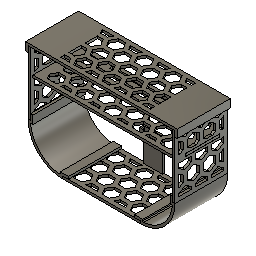
carcasa_abeja v3 (Autodesk Fusion 360 design; units mm, degrees)
Autodesk Fusion 360 part; units mm, degrees
(part 1 of 3)
sketch "Boceto1" plane through (0, 0, 0) normal (0, 1, 0) x (1, 0, 0)
  line L0 (0, 0) -> (1800, 0)
  line L1 (1800, 0) -> (1800, -650)
  line L2 (1800, -650) -> (0, -650)
  line L3 (0, -650) -> (0, 0)
  dimension "d1" = 650
  dimension "d2" = 1800
  constraint horizontal L0
  constraint vertical L1
  constraint horizontal L2
  constraint vertical L3
  constraint coincident L0.start L3.end
  measures "d1" distance of L0.end L1.end
  measures "d2" distance of L1.end L2.end
extrude "Extruir1" add sketch "Boceto1" along normal blind 30 makes body 1
sketch "Boceto3" plane through (0, 0, 0) normal (0, -1, 0) x (1, 0, 0)
  line L0 (0, 650) -> (0, 0)
  line L1 (0, 0) -> (1800, 0) construction
  line L2 (1800, 0) -> (1800, 650)
  line L3 (50, 50) -> (1750, 50)
  line L4 (1750, 50) -> (1750, 600)
  line L5 (1750, 600) -> (50, 600)
  line L6 (50, 600) -> (50, 50)
  line L7 (900, 50) -> (900, 600) construction
  line L8 (986.6025, 325) -> (943.3013, 400)
  line L9 (943.3013, 400) -> (856.6987, 400)
  line L10 (856.6987, 400) -> (813.3975, 325)
  line L11 (813.3975, 325) -> (856.6987, 250)
  line L12 (856.6987, 250) -> (943.3013, 250)
  line L13 (943.3013, 250) -> (986.6025, 325)
  line L14 (900, 325) -> (964.9519, 362.5) construction
  line L15 (1636.1216, 0) -> (1549.5191, 0) construction
  line L16 (1722.7241, 100) -> (1693.8566, 50)
  line L17 (1289.7114, 0) -> (1203.1089, 0) construction
  line L18 (1491.784, 50) -> (1462.9165, 100)
  line L19 (1376.314, 100) -> (1347.4465, 50)
  line L20 (1462.9165, 100) -> (1376.314, 100)
  line L21 (1506.2178, 125) -> (1549.5191, 50)
  line L22 (1549.5191, 50) -> (1636.1216, 50) construction
  line L23 (1636.1216, 50) -> (1679.4229, 125)
  line L24 (1679.4229, 125) -> (1636.1216, 200)
  line L25 (1549.5191, 200) -> (1506.2178, 125)
  line L26 (1636.1216, 200) -> (1549.5191, 200)
  line L27 (1679.4229, 225) -> (1722.7241, 150)
  line L28 (1722.7241, 300) -> (1679.4229, 225)
  line L29 (943.3013, 0) -> (856.6987, 0) construction
  line L30 (1145.3739, 50) -> (1116.5064, 100)
  line L31 (1029.9038, 100) -> (1001.0363, 50)
  line L32 (1116.5064, 100) -> (1029.9038, 100)
  line L33 (1159.8076, 125) -> (1203.1089, 50)
  line L34 (1203.1089, 50) -> (1289.7114, 50) construction
  line L35 (1289.7114, 50) -> (1333.0127, 125)
  line L36 (1333.0127, 125) -> (1289.7114, 200)
  line L37 (1203.1089, 200) -> (1159.8076, 125)
  line L38 (1289.7114, 200) -> (1203.1089, 200)
  line L39 (1333.0127, 225) -> (1376.314, 150)
  line L40 (1376.314, 150) -> (1462.9165, 150)
  line L41 (1462.9165, 150) -> (1506.2178, 225)
  line L42 (1506.2178, 225) -> (1462.9165, 300)
  line L43 (1376.314, 300) -> (1333.0127, 225)
  line L44 (1462.9165, 300) -> (1376.314, 300)
  line L45 (1506.2178, 325) -> (1549.5191, 250)
  line L46 (1549.5191, 250) -> (1636.1216, 250)
  line L47 (1636.1216, 250) -> (1679.4229, 325)
  line L48 (1679.4229, 325) -> (1636.1216, 400)
  line L49 (1549.5191, 400) -> (1506.2178, 325)
  line L50 (1636.1216, 400) -> (1549.5191, 400)
  line L51 (1679.4229, 425) -> (1722.7241, 350)
  line L52 (1722.7241, 500) -> (1679.4229, 425)
  line L53 (596.8911, 0) -> (510.2886, 0) construction
  line L54 (798.9637, 50) -> (770.0962, 100)
  line L55 (683.4936, 100) -> (654.6261, 50)
  line L56 (770.0962, 100) -> (683.4936, 100)
  line L57 (813.3975, 125) -> (856.6987, 50)
  line L58 (856.6987, 50) -> (943.3013, 50) construction
  line L59 (943.3013, 50) -> (986.6025, 125)
  line L60 (986.6025, 125) -> (943.3013, 200)
  line L61 (856.6987, 200) -> (813.3975, 125)
  line L62 (943.3013, 200) -> (856.6987, 200)
  line L63 (986.6025, 225) -> (1029.9038, 150)
  line L64 (1029.9038, 150) -> (1116.5064, 150)
  line L65 (1116.5064, 150) -> (1159.8076, 225)
  line L66 (1159.8076, 225) -> (1116.5064, 300)
  line L67 (1029.9038, 300) -> (986.6025, 225)
  line L68 (1116.5064, 300) -> (1029.9038, 300)
  line L69 (1159.8076, 325) -> (1203.1089, 250)
  line L70 (1203.1089, 250) -> (1289.7114, 250)
  line L71 (1289.7114, 250) -> (1333.0127, 325)
  line L72 (1333.0127, 325) -> (1289.7114, 400)
  line L73 (1203.1089, 400) -> (1159.8076, 325)
  line L74 (1289.7114, 400) -> (1203.1089, 400)
  line L75 (1333.0127, 425) -> (1376.314, 350)
  line L76 (1376.314, 350) -> (1462.9165, 350)
  line L77 (1462.9165, 350) -> (1506.2178, 425)
  line L78 (1506.2178, 425) -> (1462.9165, 500)
  line L79 (1376.314, 500) -> (1333.0127, 425)
  line L80 (1462.9165, 500) -> (1376.314, 500)
  line L81 (1506.2178, 525) -> (1549.5191, 450)
  line L82 (1549.5191, 450) -> (1636.1216, 450)
  line L83 (1636.1216, 450) -> (1679.4229, 525)
  line L84 (1679.4229, 525) -> (1636.1216, 600)
  line L85 (1549.5191, 600) -> (1506.2178, 525)
  line L86 (1636.1216, 600) -> (1549.5191, 600)
  line L87 (1693.8566, 600) -> (1722.7241, 550)
  line L88 (250.4809, 0) -> (163.8784, 0) construction
  line L89 (452.5535, 50) -> (423.686, 100)
  line L90 (337.0835, 100) -> (308.216, 50)
  line L91 (423.686, 100) -> (337.0835, 100)
  line L92 (466.9873, 125) -> (510.2886, 50)
  line L93 (510.2886, 50) -> (596.8911, 50) construction
  line L94 (596.8911, 50) -> (640.1924, 125)
  line L95 (640.1924, 125) -> (596.8911, 200)
  line L96 (510.2886, 200) -> (466.9873, 125)
  line L97 (596.8911, 200) -> (510.2886, 200)
  line L98 (640.1924, 225) -> (683.4936, 150)
  line L99 (683.4936, 150) -> (770.0962, 150)
  line L100 (770.0962, 150) -> (813.3975, 225)
  line L101 (813.3975, 225) -> (770.0962, 300)
  line L102 (683.4936, 300) -> (640.1924, 225)
  line L103 (770.0962, 300) -> (683.4936, 300)
  line L104 (986.6025, 425) -> (1029.9038, 350)
  line L105 (1029.9038, 350) -> (1116.5064, 350)
  line L106 (1116.5064, 350) -> (1159.8076, 425)
  line L107 (1159.8076, 425) -> (1116.5064, 500)
  line L108 (1029.9038, 500) -> (986.6025, 425)
  line L109 (1116.5064, 500) -> (1029.9038, 500)
  line L110 (1159.8076, 525) -> (1203.1089, 450)
  line L111 (1203.1089, 450) -> (1289.7114, 450)
  line L112 (1289.7114, 450) -> (1333.0127, 525)
  line L113 (1333.0127, 525) -> (1289.7114, 600)
  line L114 (1203.1089, 600) -> (1159.8076, 525)
  line L115 (1289.7114, 600) -> (1203.1089, 600)
  line L116 (1347.4465, 600) -> (1376.314, 550)
  line L117 (1376.314, 550) -> (1462.9165, 550)
  line L118 (1462.9165, 550) -> (1491.784, 600)
  line L119 (106.1434, 50) -> (77.2759, 100)
  line L120 (120.5771, 125) -> (163.8784, 50)
  line L121 (163.8784, 50) -> (250.4809, 50) construction
  line L122 (250.4809, 50) -> (293.7822, 125)
  line L123 (293.7822, 125) -> (250.4809, 200)
  line L124 (163.8784, 200) -> (120.5771, 125)
  line L125 (250.4809, 200) -> (163.8784, 200)
  line L126 (293.7822, 225) -> (337.0835, 150)
  line L127 (337.0835, 150) -> (423.686, 150)
  line L128 (423.686, 150) -> (466.9873, 225)
  line L129 (466.9873, 225) -> (423.686, 300)
  line L130 (337.0835, 300) -> (293.7822, 225)
  line L131 (423.686, 300) -> (337.0835, 300)
  line L132 (466.9873, 325) -> (510.2886, 250)
  line L133 (510.2886, 250) -> (596.8911, 250)
  line L134 (596.8911, 250) -> (640.1924, 325)
  line L135 (640.1924, 325) -> (596.8911, 400)
  line L136 (510.2886, 400) -> (466.9873, 325)
  line L137 (596.8911, 400) -> (510.2886, 400)
  line L138 (640.1924, 425) -> (683.4936, 350)
  line L139 (683.4936, 350) -> (770.0962, 350)
  line L140 (770.0962, 350) -> (813.3975, 425)
  line L141 (813.3975, 425) -> (770.0962, 500)
  line L142 (683.4936, 500) -> (640.1924, 425)
  line L143 (770.0962, 500) -> (683.4936, 500)
  line L144 (813.3975, 525) -> (856.6987, 450)
  line L145 (856.6987, 450) -> (943.3013, 450)
  line L146 (943.3013, 450) -> (986.6025, 525)
  line L147 (986.6025, 525) -> (943.3013, 600)
  line L148 (856.6987, 600) -> (813.3975, 525)
  line L149 (943.3013, 600) -> (856.6987, 600)
  line L150 (1001.0363, 600) -> (1029.9038, 550)
  line L151 (1029.9038, 550) -> (1116.5064, 550)
  line L152 (1116.5064, 550) -> (1145.3739, 600)
  line L153 (77.2759, 150) -> (120.5771, 225)
  line L154 (120.5771, 225) -> (77.2759, 300)
  line L155 (120.5771, 325) -> (163.8784, 250)
  line L156 (163.8784, 250) -> (250.4809, 250)
  line L157 (250.4809, 250) -> (293.7822, 325)
  line L158 (293.7822, 325) -> (250.4809, 400)
  line L159 (163.8784, 400) -> (120.5771, 325)
  line L160 (250.4809, 400) -> (163.8784, 400)
  line L161 (293.7822, 425) -> (337.0835, 350)
  line L162 (337.0835, 350) -> (423.686, 350)
  line L163 (423.686, 350) -> (466.9873, 425)
  line L164 (466.9873, 425) -> (423.686, 500)
  line L165 (337.0835, 500) -> (293.7822, 425)
  line L166 (423.686, 500) -> (337.0835, 500)
  line L167 (466.9873, 525) -> (510.2886, 450)
  line L168 (510.2886, 450) -> (596.8911, 450)
  line L169 (596.8911, 450) -> (640.1924, 525)
  line L170 (640.1924, 525) -> (596.8911, 600)
  line L171 (510.2886, 600) -> (466.9873, 525)
  line L172 (596.8911, 600) -> (510.2886, 600)
  line L173 (654.6261, 600) -> (683.4936, 550)
  line L174 (683.4936, 550) -> (770.0962, 550)
  line L175 (770.0962, 550) -> (798.9637, 600)
  line L176 (77.2759, 350) -> (120.5771, 425)
  line L177 (120.5771, 425) -> (77.2759, 500)
  line L178 (120.5771, 525) -> (163.8784, 450)
  line L179 (163.8784, 450) -> (250.4809, 450)
  line L180 (250.4809, 450) -> (293.7822, 525)
  line L181 (293.7822, 525) -> (250.4809, 600)
  line L182 (163.8784, 600) -> (120.5771, 525)
  line L183 (250.4809, 600) -> (163.8784, 600)
  line L184 (308.216, 600) -> (337.0835, 550)
  line L185 (337.0835, 550) -> (423.686, 550)
  line L186 (423.686, 550) -> (452.5535, 600)
  line L187 (77.2759, 550) -> (106.1434, 600)
  line L188 (77.2759, 500) -> (50, 500)
  line L189 (0, 500) -> (-9.3267, 500)
  line L190 (-9.3267, 350) -> (0, 350)
  line L191 (50, 350) -> (77.2759, 350)
  line L192 (-9.3267, 550) -> (0, 550)
  line L193 (50, 550) -> (77.2759, 550)
  line L194 (1722.7241, 550) -> (1750, 550)
  line L195 (1800, 550) -> (1809.3267, 550)
  line L196 (1809.3267, 500) -> (1800, 500)
  line L197 (1750, 500) -> (1722.7241, 500)
  line L198 (1722.7241, 350) -> (1750, 350)
  line L199 (1800, 350) -> (1809.3267, 350)
  line L200 (1809.3267, 300) -> (1800, 300)
  line L201 (1750, 300) -> (1722.7241, 300)
  line L202 (1722.7241, 150) -> (1750, 150)
  line L203 (1800, 150) -> (1809.3267, 150)
  line L204 (1809.3267, 100) -> (1800, 100)
  line L205 (1750, 100) -> (1722.7241, 100)
  line L206 (77.2759, 100) -> (50, 100)
  line L207 (0, 100) -> (-9.3267, 100)
  line L208 (-9.3267, 150) -> (0, 150)
  line L209 (50, 150) -> (77.2759, 150)
  line L210 (77.2759, 300) -> (50, 300)
  line L211 (0, 300) -> (-9.3267, 300)
  point P0 (900, 325)
  dimension "d15" = 200
  dimension "d16" = 200
  dimension "d17" = 150
  constraint midpoint L3 L7.start
  constraint midpoint L5 L7.end
  constraint midpoint L7 P0
  constraint parallel L3 L12
  constraint coincident P0 L14.start
  constraint midpoint L8 L14.end
  constraint coincident L6 L188.end
  constraint coincident L0 L189.start
  constraint collinear L188 L189
  constraint coincident L0 L190.end
  constraint coincident L6 L191.start
  constraint collinear L190 L191
  constraint coincident L0 L192.end
  constraint coincident L6 L193.start
  constraint collinear L192 L193
  constraint coincident L5 L187.end
  constraint coincident L5 L184.start
  constraint coincident L5 L186.end
  constraint coincident L5 L173.start
  constraint coincident L5 L175.end
  constraint coincident L5 L150.start
  constraint coincident L5 L152.end
  constraint coincident L5 L116.start
  constraint coincident L5 L118.end
  constraint coincident L5 L87.start
  constraint coincident L4 L194.end
  constraint coincident L2 L195.start
  constraint collinear L194 L195
  constraint coincident L2 L196.end
  constraint coincident L4 L197.start
  constraint collinear L196 L197
  constraint coincident L4 L198.end
  constraint coincident L2 L199.start
  constraint collinear L198 L199
  constraint coincident L2 L200.end
  constraint coincident L4 L201.start
  constraint collinear L200 L201
  constraint coincident L4 L202.end
  constraint coincident L2 L203.start
  constraint collinear L202 L203
  constraint coincident L2 L204.end
  constraint coincident L4 L205.start
  constraint collinear L204 L205
  constraint coincident L3 L16.end
  constraint coincident L3 L18.start
  constraint coincident L3 L19.end
  constraint coincident L3 L30.start
  constraint coincident L3 L31.end
  constraint coincident L3 L54.start
  constraint coincident L3 L55.end
  constraint coincident L3 L89.start
  constraint coincident L3 L90.end
  constraint coincident L3 L119.start
  constraint coincident L6 L206.end
  constraint coincident L0 L207.start
  constraint collinear L206 L207
  constraint coincident L0 L208.end
  constraint coincident L6 L209.start
  constraint collinear L208 L209
  constraint coincident L6 L210.end
  constraint coincident L0 L211.start
  constraint collinear L210 L211
  measures "d17" distance of L8.end L12.end
extrude "Extruir2" cut sketch "Boceto3" against normal blind 300 contours L3 L6 L119 L206 | L3 L120 L122 L123 L124 L125 | L6 L153 L154 L209 L210 | L3 L89 L90 L91 | L6 L176 L177 L188 L191 | L3 L92 L94 L95 L96 L97 | L5 L6 L187 L193 | L3 L54 L55 L56 | L5 L178 L179 L180 L181 L182 L183 | L3 L57 L59 L60 L61 L62 | L5 L184 L185 L186 | L3 L30 L31 L32 | L5 L167 L168 L169 L170 L171 L172 | L3 L33 L35 L36 L37 L38 | L5 L173 L174 L175 | L3 L18 L19 L20 | L5 L144 L145 L146 L147 L148 L149 | L3 L21 L23 L24 L25 L26 | L5 L150 L151 L152 | L3 L4 L16 L205 | L5 L110 L111 L112 L113 L114 L115 | L4 L27 L28 L201 L202 | L5 L116 L117 L118 | L4 L51 L52 L197 L198 | L5 L81 L82 L83 L84 L85 L86 | L4 L5 L87 L194 | L8 L9 L10 L11 L12 L13 | L39 L40 L41 L42 L43 L44 | L45 L46 L47 L48 L49 L50 | L63 L64 L65 L66 L67 L68 | L69 L70 L71 L72 L73 L74 | L75 L76 L77 L78 L79 L80 | L98 L99 L100 L101 L102 L103 | L104 L105 L106 L107 L108 L109 | L126 L127 L128 L129 L130 L131 | L132 L133 L134 L135 L136 L137 | L138 L139 L140 L141 L142 L143 | L155 L156 L157 L158 L159 L160 | L161 L162 L163 L164 L165 L166 bodies 1
sketch "Boceto4" plane through (0, 30, 0) normal (0, 1, 0) x (-1, 0, 0)
  line L0 (-1549.5191, 200) -> (-1506.2178, 125)
  line L1 (-1506.2178, 125) -> (-1549.5191, 50)
  line L2 (-1549.5191, 50) -> (-1636.1216, 50)
  line L3 (-1636.1216, 50) -> (-1679.4229, 125)
  line L4 (-1679.4229, 125) -> (-1636.1216, 200)
  line L5 (-1636.1216, 200) -> (-1549.5191, 200)
  line L6 (-1750, 550) -> (-1750, 600)
  line L7 (-1750, 600) -> (-1693.8566, 600)
  line L8 (-1693.8566, 600) -> (-1722.7241, 550)
  line L9 (-1722.7241, 550) -> (-1750, 550)
  line L10 (-1376.314, 300) -> (-1333.0127, 225)
  line L11 (-1333.0127, 225) -> (-1376.314, 150)
  line L12 (-1376.314, 150) -> (-1462.9165, 150)
  line L13 (-1462.9165, 150) -> (-1506.2178, 225)
  line L14 (-1506.2178, 225) -> (-1462.9165, 300)
  line L15 (-1462.9165, 300) -> (-1376.314, 300)
  line L16 (-1203.1089, 600) -> (-1159.8076, 525)
  line L17 (-1159.8076, 525) -> (-1203.1089, 450)
  line L18 (-1203.1089, 450) -> (-1289.7114, 450)
  line L19 (-1289.7114, 450) -> (-1333.0127, 525)
  line L20 (-1333.0127, 525) -> (-1289.7114, 600)
  line L21 (-1289.7114, 600) -> (-1203.1089, 600)
  line L22 (-856.6987, 200) -> (-813.3975, 125)
  line L23 (-813.3975, 125) -> (-856.6987, 50)
  line L24 (-856.6987, 50) -> (-943.3013, 50)
  line L25 (-943.3013, 50) -> (-986.6025, 125)
  line L26 (-986.6025, 125) -> (-943.3013, 200)
  line L27 (-943.3013, 200) -> (-856.6987, 200)
  line L28 (-856.6987, 600) -> (-813.3975, 525)
  line L29 (-813.3975, 525) -> (-856.6987, 450)
  line L30 (-856.6987, 450) -> (-943.3013, 450)
  line L31 (-943.3013, 450) -> (-986.6025, 525)
  line L32 (-986.6025, 525) -> (-943.3013, 600)
  line L33 (-943.3013, 600) -> (-856.6987, 600)
  line L34 (-510.2886, 400) -> (-466.9873, 325)
  line L35 (-466.9873, 325) -> (-510.2886, 250)
  line L36 (-510.2886, 250) -> (-596.8911, 250)
  line L37 (-596.8911, 250) -> (-640.1924, 325)
  line L38 (-640.1924, 325) -> (-596.8911, 400)
  line L39 (-596.8911, 400) -> (-510.2886, 400)
  line L40 (-163.8784, 400) -> (-120.5771, 325)
  line L41 (-120.5771, 325) -> (-163.8784, 250)
  line L42 (-163.8784, 250) -> (-250.4809, 250)
  line L43 (-250.4809, 250) -> (-293.7822, 325)
  line L44 (-293.7822, 325) -> (-250.4809, 400)
  line L45 (-250.4809, 400) -> (-163.8784, 400)
  line L46 (-77.2759, 350) -> (-120.5771, 425)
  line L47 (-120.5771, 425) -> (-77.2759, 500)
  line L48 (-77.2759, 500) -> (-50, 500)
  line L49 (-50, 500) -> (-50, 350)
  line L50 (-50, 350) -> (-77.2759, 350)
  line L51 (-163.8784, 600) -> (-120.5771, 525)
  line L52 (-120.5771, 525) -> (-163.8784, 450)
  line L53 (-163.8784, 450) -> (-250.4809, 450)
  line L54 (-250.4809, 450) -> (-293.7822, 525)
  line L55 (-293.7822, 525) -> (-250.4809, 600)
  line L56 (-250.4809, 600) -> (-163.8784, 600)
  line L57 (-77.2759, 550) -> (-106.1434, 600)
  line L58 (-106.1434, 600) -> (-50, 600)
  line L59 (-50, 600) -> (-50, 550)
  line L60 (-50, 550) -> (-77.2759, 550)
  line L61 (-163.8784, 200) -> (-120.5771, 125)
  line L62 (-120.5771, 125) -> (-163.8784, 50)
  line L63 (-163.8784, 50) -> (-250.4809, 50)
  line L64 (-250.4809, 50) -> (-293.7822, 125)
  line L65 (-293.7822, 125) -> (-250.4809, 200)
  line L66 (-250.4809, 200) -> (-163.8784, 200)
  line L67 (-510.2886, 200) -> (-466.9873, 125)
  line L68 (-466.9873, 125) -> (-510.2886, 50)
  line L69 (-510.2886, 50) -> (-596.8911, 50)
  line L70 (-596.8911, 50) -> (-640.1924, 125)
  line L71 (-640.1924, 125) -> (-596.8911, 200)
  line L72 (-596.8911, 200) -> (-510.2886, 200)
  line L73 (-683.4936, 500) -> (-640.1924, 425)
  line L74 (-640.1924, 425) -> (-683.4936, 350)
  line L75 (-683.4936, 350) -> (-770.0962, 350)
  line L76 (-770.0962, 350) -> (-813.3975, 425)
  line L77 (-813.3975, 425) -> (-770.0962, 500)
  line L78 (-770.0962, 500) -> (-683.4936, 500)
  line L79 (-683.4936, 100) -> (-654.6261, 50)
  line L80 (-654.6261, 50) -> (-798.9637, 50)
  line L81 (-798.9637, 50) -> (-770.0962, 100)
  line L82 (-770.0962, 100) -> (-683.4936, 100)
  line L83 (-1145.3739, 600) -> (-1001.0363, 600)
  line L84 (-1001.0363, 600) -> (-1029.9038, 550)
  line L85 (-1029.9038, 550) -> (-1116.5064, 550)
  line L86 (-1116.5064, 550) -> (-1145.3739, 600)
  line L87 (-1203.1089, 200) -> (-1159.8076, 125)
  line L88 (-1159.8076, 125) -> (-1203.1089, 50)
  line L89 (-1203.1089, 50) -> (-1289.7114, 50)
  line L90 (-1289.7114, 50) -> (-1333.0127, 125)
  line L91 (-1333.0127, 125) -> (-1289.7114, 200)
  line L92 (-1289.7114, 200) -> (-1203.1089, 200)
  line L93 (-1549.5191, 600) -> (-1506.2178, 525)
  line L94 (-1506.2178, 525) -> (-1549.5191, 450)
  line L95 (-1549.5191, 450) -> (-1636.1216, 450)
  line L96 (-1636.1216, 450) -> (-1679.4229, 525)
  line L97 (-1679.4229, 525) -> (-1636.1216, 600)
  line L98 (-1636.1216, 600) -> (-1549.5191, 600)
  line L99 (-1376.314, 100) -> (-1347.4465, 50)
  line L100 (-1347.4465, 50) -> (-1491.784, 50)
  line L101 (-1491.784, 50) -> (-1462.9165, 100)
  line L102 (-1462.9165, 100) -> (-1376.314, 100)
  line L103 (-1750, 150) -> (-1750, 300)
  line L104 (-1750, 300) -> (-1722.7241, 300)
  line L105 (-1722.7241, 300) -> (-1679.4229, 225)
  line L106 (-1679.4229, 225) -> (-1722.7241, 150)
  line L107 (-1722.7241, 150) -> (-1750, 150)
  line L108 (-1750, 350) -> (-1750, 500)
  line L109 (-1750, 500) -> (-1722.7241, 500)
  line L110 (-1722.7241, 500) -> (-1679.4229, 425)
  line L111 (-1679.4229, 425) -> (-1722.7241, 350)
  line L112 (-1722.7241, 350) -> (-1750, 350)
  line L113 (-1376.314, 500) -> (-1333.0127, 425)
  line L114 (-1333.0127, 425) -> (-1376.314, 350)
  line L115 (-1376.314, 350) -> (-1462.9165, 350)
  line L116 (-1462.9165, 350) -> (-1506.2178, 425)
  line L117 (-1506.2178, 425) -> (-1462.9165, 500)
  line L118 (-1462.9165, 500) -> (-1376.314, 500)
  line L119 (-1203.1089, 400) -> (-1159.8076, 325)
  line L120 (-1159.8076, 325) -> (-1203.1089, 250)
  line L121 (-1203.1089, 250) -> (-1289.7114, 250)
  line L122 (-1289.7114, 250) -> (-1333.0127, 325)
  line L123 (-1333.0127, 325) -> (-1289.7114, 400)
  line L124 (-1289.7114, 400) -> (-1203.1089, 400)
  line L125 (-1029.9038, 300) -> (-986.6025, 225)
  line L126 (-986.6025, 225) -> (-1029.9038, 150)
  line L127 (-1029.9038, 150) -> (-1116.5064, 150)
  line L128 (-1116.5064, 150) -> (-1159.8076, 225)
  line L129 (-1159.8076, 225) -> (-1116.5064, 300)
  line L130 (-1116.5064, 300) -> (-1029.9038, 300)
  line L131 (-683.4936, 300) -> (-640.1924, 225)
  line L132 (-640.1924, 225) -> (-683.4936, 150)
  line L133 (-683.4936, 150) -> (-770.0962, 150)
  line L134 (-770.0962, 150) -> (-813.3975, 225)
  line L135 (-813.3975, 225) -> (-770.0962, 300)
  line L136 (-770.0962, 300) -> (-683.4936, 300)
  line L137 (-510.2886, 600) -> (-466.9873, 525)
  line L138 (-466.9873, 525) -> (-510.2886, 450)
  line L139 (-510.2886, 450) -> (-596.8911, 450)
  line L140 (-596.8911, 450) -> (-640.1924, 525)
  line L141 (-640.1924, 525) -> (-596.8911, 600)
  line L142 (-596.8911, 600) -> (-510.2886, 600)
  line L143 (-337.0835, 300) -> (-293.7822, 225)
  line L144 (-293.7822, 225) -> (-337.0835, 150)
  line L145 (-337.0835, 150) -> (-423.686, 150)
  line L146 (-423.686, 150) -> (-466.9873, 225)
  line L147 (-466.9873, 225) -> (-423.686, 300)
  line L148 (-423.686, 300) -> (-337.0835, 300)
  line L149 (-50, 300) -> (-50, 150)
  line L150 (-50, 150) -> (-77.2759, 150)
  line L151 (-77.2759, 150) -> (-120.5771, 225)
  line L152 (-120.5771, 225) -> (-77.2759, 300)
  line L153 (-77.2759, 300) -> (-50, 300)
  line L154 (-337.0835, 500) -> (-293.7822, 425)
  line L155 (-293.7822, 425) -> (-337.0835, 350)
  line L156 (-337.0835, 350) -> (-423.686, 350)
  line L157 (-423.686, 350) -> (-466.9873, 425)
  line L158 (-466.9873, 425) -> (-423.686, 500)
  line L159 (-423.686, 500) -> (-337.0835, 500)
  line L160 (-452.5535, 600) -> (-308.216, 600)
  line L161 (-308.216, 600) -> (-337.0835, 550)
  line L162 (-337.0835, 550) -> (-423.686, 550)
  line L163 (-423.686, 550) -> (-452.5535, 600)
  line L164 (-50, 100) -> (-50, 50)
  line L165 (-50, 50) -> (-106.1434, 50)
  line L166 (-106.1434, 50) -> (-77.2759, 100)
  line L167 (-77.2759, 100) -> (-50, 100)
  line L168 (-337.0835, 100) -> (-308.216, 50)
  line L169 (-308.216, 50) -> (-452.5535, 50)
  line L170 (-452.5535, 50) -> (-423.686, 100)
  line L171 (-423.686, 100) -> (-337.0835, 100)
  line L172 (-798.9637, 600) -> (-654.6261, 600)
  line L173 (-654.6261, 600) -> (-683.4936, 550)
  line L174 (-683.4936, 550) -> (-770.0962, 550)
  line L175 (-770.0962, 550) -> (-798.9637, 600)
  line L176 (-986.6025, 325) -> (-943.3013, 400)
  line L177 (-943.3013, 400) -> (-856.6987, 400)
  line L178 (-856.6987, 400) -> (-813.3975, 325)
  line L179 (-813.3975, 325) -> (-856.6987, 250)
  line L180 (-856.6987, 250) -> (-943.3013, 250)
  line L181 (-943.3013, 250) -> (-986.6025, 325)
  line L182 (-1029.9038, 500) -> (-986.6025, 425)
  line L183 (-986.6025, 425) -> (-1029.9038, 350)
  line L184 (-1029.9038, 350) -> (-1116.5064, 350)
  line L185 (-1116.5064, 350) -> (-1159.8076, 425)
  line L186 (-1159.8076, 425) -> (-1116.5064, 500)
  line L187 (-1116.5064, 500) -> (-1029.9038, 500)
  line L188 (-1029.9038, 100) -> (-1001.0363, 50)
  line L189 (-1001.0363, 50) -> (-1145.3739, 50)
  line L190 (-1145.3739, 50) -> (-1116.5064, 100)
  line L191 (-1116.5064, 100) -> (-1029.9038, 100)
  line L192 (-1491.784, 600) -> (-1347.4465, 600)
  line L193 (-1347.4465, 600) -> (-1376.314, 550)
  line L194 (-1376.314, 550) -> (-1462.9165, 550)
  line L195 (-1462.9165, 550) -> (-1491.784, 600)
  line L196 (-1549.5191, 400) -> (-1506.2178, 325)
  line L197 (-1506.2178, 325) -> (-1549.5191, 250)
  line L198 (-1549.5191, 250) -> (-1636.1216, 250)
  line L199 (-1636.1216, 250) -> (-1679.4229, 325)
  line L200 (-1679.4229, 325) -> (-1636.1216, 400)
  line L201 (-1636.1216, 400) -> (-1549.5191, 400)
  line L202 (-1722.7241, 100) -> (-1693.8566, 50)
  line L203 (-1693.8566, 50) -> (-1750, 50)
  line L204 (-1750, 50) -> (-1750, 100)
  line L205 (-1750, 100) -> (-1722.7241, 100)
  line L206 (0, 650) -> (-1800, 650)
  line L207 (-1800, 650) -> (-1800, 0)
  line L208 (-1800, 0) -> (0, 0)
  line L209 (0, 0) -> (0, 650)
scale "Escala1" factor 0.1 about (986.6025, 30, 325) bodies 1
sketch "Boceto5" plane through (0, 30, 0) normal (0, 1, 0) x (-1, 0, 0)
  line L0 (-1042.8942, 312.5) -> (-1038.5641, 305)
  line L1 (-1038.5641, 305) -> (-1042.8942, 297.5)
  line L2 (-1042.8942, 297.5) -> (-1051.5544, 297.5)
  line L3 (-1051.5544, 297.5) -> (-1055.8846, 305)
  line L4 (-1055.8846, 305) -> (-1051.5544, 312.5)
  line L5 (-1051.5544, 312.5) -> (-1042.8942, 312.5)
  line L6 (-1062.9423, 347.5) -> (-1062.9423, 352.5)
  line L7 (-1062.9423, 352.5) -> (-1057.3279, 352.5)
  line L8 (-1057.3279, 352.5) -> (-1060.2147, 347.5)
  line L9 (-1060.2147, 347.5) -> (-1062.9423, 347.5)
  line L10 (-1025.5737, 322.5) -> (-1021.2436, 315)
  line L11 (-1021.2436, 315) -> (-1025.5737, 307.5)
  line L12 (-1025.5737, 307.5) -> (-1034.2339, 307.5)
  line L13 (-1034.2339, 307.5) -> (-1038.5641, 315)
  line L14 (-1038.5641, 315) -> (-1034.2339, 322.5)
  line L15 (-1034.2339, 322.5) -> (-1025.5737, 322.5)
  line L16 (-1008.2532, 352.5) -> (-1003.923, 345)
  line L17 (-1003.923, 345) -> (-1008.2532, 337.5)
  line L18 (-1008.2532, 337.5) -> (-1016.9134, 337.5)
  line L19 (-1016.9134, 337.5) -> (-1021.2436, 345)
  line L20 (-1021.2436, 345) -> (-1016.9134, 352.5)
  line L21 (-1016.9134, 352.5) -> (-1008.2532, 352.5)
  line L22 (-973.6122, 312.5) -> (-969.282, 305)
  line L23 (-969.282, 305) -> (-973.6122, 297.5)
  line L24 (-973.6122, 297.5) -> (-982.2724, 297.5)
  line L25 (-982.2724, 297.5) -> (-986.6025, 305)
  line L26 (-986.6025, 305) -> (-982.2724, 312.5)
  line L27 (-982.2724, 312.5) -> (-973.6122, 312.5)
  line L28 (-973.6122, 352.5) -> (-969.282, 345)
  line L29 (-969.282, 345) -> (-973.6122, 337.5)
  line L30 (-973.6122, 337.5) -> (-982.2724, 337.5)
  line L31 (-982.2724, 337.5) -> (-986.6025, 345)
  line L32 (-986.6025, 345) -> (-982.2724, 352.5)
  line L33 (-982.2724, 352.5) -> (-973.6122, 352.5)
  line L34 (-938.9711, 332.5) -> (-934.641, 325)
  line L35 (-934.641, 325) -> (-938.9711, 317.5)
  line L36 (-938.9711, 317.5) -> (-947.6314, 317.5)
  line L37 (-947.6314, 317.5) -> (-951.9615, 325)
  line L38 (-951.9615, 325) -> (-947.6314, 332.5)
  line L39 (-947.6314, 332.5) -> (-938.9711, 332.5)
  line L40 (-904.3301, 332.5) -> (-900, 325)
  line L41 (-900, 325) -> (-904.3301, 317.5)
  line L42 (-904.3301, 317.5) -> (-912.9904, 317.5)
  line L43 (-912.9904, 317.5) -> (-917.3205, 325)
  line L44 (-917.3205, 325) -> (-912.9904, 332.5)
  line L45 (-912.9904, 332.5) -> (-904.3301, 332.5)
  line L46 (-895.6699, 327.5) -> (-900, 335)
  line L47 (-900, 335) -> (-895.6699, 342.5)
  line L48 (-895.6699, 342.5) -> (-892.9423, 342.5)
  line L49 (-892.9423, 342.5) -> (-892.9423, 327.5)
  line L50 (-892.9423, 327.5) -> (-895.6699, 327.5)
  line L51 (-904.3301, 352.5) -> (-900, 345)
  line L52 (-900, 345) -> (-904.3301, 337.5)
  line L53 (-904.3301, 337.5) -> (-912.9904, 337.5)
  line L54 (-912.9904, 337.5) -> (-917.3205, 345)
  line L55 (-917.3205, 345) -> (-912.9904, 352.5)
  line L56 (-912.9904, 352.5) -> (-904.3301, 352.5)
  line L57 (-895.6699, 347.5) -> (-898.5566, 352.5)
  line L58 (-898.5566, 352.5) -> (-892.9423, 352.5)
  line L59 (-892.9423, 352.5) -> (-892.9423, 347.5)
  line L60 (-892.9423, 347.5) -> (-895.6699, 347.5)
  line L61 (-904.3301, 312.5) -> (-900, 305)
  line L62 (-900, 305) -> (-904.3301, 297.5)
  line L63 (-904.3301, 297.5) -> (-912.9904, 297.5)
  line L64 (-912.9904, 297.5) -> (-917.3205, 305)
  line L65 (-917.3205, 305) -> (-912.9904, 312.5)
  line L66 (-912.9904, 312.5) -> (-904.3301, 312.5)
  line L67 (-938.9711, 312.5) -> (-934.641, 305)
  line L68 (-934.641, 305) -> (-938.9711, 297.5)
  line L69 (-938.9711, 297.5) -> (-947.6314, 297.5)
  line L70 (-947.6314, 297.5) -> (-951.9615, 305)
  line L71 (-951.9615, 305) -> (-947.6314, 312.5)
  line L72 (-947.6314, 312.5) -> (-938.9711, 312.5)
  line L73 (-956.2917, 342.5) -> (-951.9615, 335)
  line L74 (-951.9615, 335) -> (-956.2917, 327.5)
  line L75 (-956.2917, 327.5) -> (-964.9519, 327.5)
  line L76 (-964.9519, 327.5) -> (-969.282, 335)
  line L77 (-969.282, 335) -> (-964.9519, 342.5)
  line L78 (-964.9519, 342.5) -> (-956.2917, 342.5)
  line L79 (-956.2917, 302.5) -> (-953.4049, 297.5)
  line L80 (-953.4049, 297.5) -> (-967.8387, 297.5)
  line L81 (-967.8387, 297.5) -> (-964.9519, 302.5)
  line L82 (-964.9519, 302.5) -> (-956.2917, 302.5)
  line L83 (-1002.4797, 352.5) -> (-988.0459, 352.5)
  line L84 (-988.0459, 352.5) -> (-990.9327, 347.5)
  line L85 (-990.9327, 347.5) -> (-999.5929, 347.5)
  line L86 (-999.5929, 347.5) -> (-1002.4797, 352.5)
  line L87 (-1008.2532, 312.5) -> (-1003.923, 305)
  line L88 (-1003.923, 305) -> (-1008.2532, 297.5)
  line L89 (-1008.2532, 297.5) -> (-1016.9134, 297.5)
  line L90 (-1016.9134, 297.5) -> (-1021.2436, 305)
  line L91 (-1021.2436, 305) -> (-1016.9134, 312.5)
  line L92 (-1016.9134, 312.5) -> (-1008.2532, 312.5)
  line L93 (-1042.8942, 352.5) -> (-1038.5641, 345)
  line L94 (-1038.5641, 345) -> (-1042.8942, 337.5)
  line L95 (-1042.8942, 337.5) -> (-1051.5544, 337.5)
  line L96 (-1051.5544, 337.5) -> (-1055.8846, 345)
  line L97 (-1055.8846, 345) -> (-1051.5544, 352.5)
  line L98 (-1051.5544, 352.5) -> (-1042.8942, 352.5)
  line L99 (-1025.5737, 302.5) -> (-1022.6869, 297.5)
  line L100 (-1022.6869, 297.5) -> (-1037.1207, 297.5)
  line L101 (-1037.1207, 297.5) -> (-1034.2339, 302.5)
  line L102 (-1034.2339, 302.5) -> (-1025.5737, 302.5)
  line L103 (-1062.9423, 307.5) -> (-1062.9423, 322.5)
  line L104 (-1062.9423, 322.5) -> (-1060.2147, 322.5)
  line L105 (-1060.2147, 322.5) -> (-1055.8846, 315)
  line L106 (-1055.8846, 315) -> (-1060.2147, 307.5)
  line L107 (-1060.2147, 307.5) -> (-1062.9423, 307.5)
  line L108 (-1062.9423, 327.5) -> (-1062.9423, 342.5)
  line L109 (-1062.9423, 342.5) -> (-1060.2147, 342.5)
  line L110 (-1060.2147, 342.5) -> (-1055.8846, 335)
  line L111 (-1055.8846, 335) -> (-1060.2147, 327.5)
  line L112 (-1060.2147, 327.5) -> (-1062.9423, 327.5)
  line L113 (-1025.5737, 342.5) -> (-1021.2436, 335)
  line L114 (-1021.2436, 335) -> (-1025.5737, 327.5)
  line L115 (-1025.5737, 327.5) -> (-1034.2339, 327.5)
  line L116 (-1034.2339, 327.5) -> (-1038.5641, 335)
  line L117 (-1038.5641, 335) -> (-1034.2339, 342.5)
  line L118 (-1034.2339, 342.5) -> (-1025.5737, 342.5)
  line L119 (-1008.2532, 332.5) -> (-1003.923, 325)
  line L120 (-1003.923, 325) -> (-1008.2532, 317.5)
  line L121 (-1008.2532, 317.5) -> (-1016.9134, 317.5)
  line L122 (-1016.9134, 317.5) -> (-1021.2436, 325)
  line L123 (-1021.2436, 325) -> (-1016.9134, 332.5)
  line L124 (-1016.9134, 332.5) -> (-1008.2532, 332.5)
  line L125 (-990.9327, 322.5) -> (-986.6025, 315)
  line L126 (-986.6025, 315) -> (-990.9327, 307.5)
  line L127 (-990.9327, 307.5) -> (-999.5929, 307.5)
  line L128 (-999.5929, 307.5) -> (-1003.923, 315)
  line L129 (-1003.923, 315) -> (-999.5929, 322.5)
  line L130 (-999.5929, 322.5) -> (-990.9327, 322.5)
  line L131 (-956.2917, 322.5) -> (-951.9615, 315)
  line L132 (-951.9615, 315) -> (-956.2917, 307.5)
  line L133 (-956.2917, 307.5) -> (-964.9519, 307.5)
  line L134 (-964.9519, 307.5) -> (-969.282, 315)
  line L135 (-969.282, 315) -> (-964.9519, 322.5)
  line L136 (-964.9519, 322.5) -> (-956.2917, 322.5)
  line L137 (-938.9711, 352.5) -> (-934.641, 345)
  line L138 (-934.641, 345) -> (-938.9711, 337.5)
  line L139 (-938.9711, 337.5) -> (-947.6314, 337.5)
  line L140 (-947.6314, 337.5) -> (-951.9615, 345)
  line L141 (-951.9615, 345) -> (-947.6314, 352.5)
  line L142 (-947.6314, 352.5) -> (-938.9711, 352.5)
  line L143 (-921.6506, 322.5) -> (-917.3205, 315)
  line L144 (-917.3205, 315) -> (-921.6506, 307.5)
  line L145 (-921.6506, 307.5) -> (-930.3109, 307.5)
  line L146 (-930.3109, 307.5) -> (-934.641, 315)
  line L147 (-934.641, 315) -> (-930.3109, 322.5)
  line L148 (-930.3109, 322.5) -> (-921.6506, 322.5)
  line L149 (-892.9423, 322.5) -> (-892.9423, 307.5)
  line L150 (-892.9423, 307.5) -> (-895.6699, 307.5)
  line L151 (-895.6699, 307.5) -> (-900, 315)
  line L152 (-900, 315) -> (-895.6699, 322.5)
  line L153 (-895.6699, 322.5) -> (-892.9423, 322.5)
  line L154 (-921.6506, 342.5) -> (-917.3205, 335)
  line L155 (-917.3205, 335) -> (-921.6506, 327.5)
  line L156 (-921.6506, 327.5) -> (-930.3109, 327.5)
  line L157 (-930.3109, 327.5) -> (-934.641, 335)
  line L158 (-934.641, 335) -> (-930.3109, 342.5)
  line L159 (-930.3109, 342.5) -> (-921.6506, 342.5)
  line L160 (-933.1976, 352.5) -> (-918.7639, 352.5)
  line L161 (-918.7639, 352.5) -> (-921.6506, 347.5)
  line L162 (-921.6506, 347.5) -> (-930.3109, 347.5)
  line L163 (-930.3109, 347.5) -> (-933.1976, 352.5)
  line L164 (-892.9423, 302.5) -> (-892.9423, 297.5)
  line L165 (-892.9423, 297.5) -> (-898.5566, 297.5)
  line L166 (-898.5566, 297.5) -> (-895.6699, 302.5)
  line L167 (-895.6699, 302.5) -> (-892.9423, 302.5)
  line L168 (-921.6506, 302.5) -> (-918.7639, 297.5)
  line L169 (-918.7639, 297.5) -> (-933.1976, 297.5)
  line L170 (-933.1976, 297.5) -> (-930.3109, 302.5)
  line L171 (-930.3109, 302.5) -> (-921.6506, 302.5)
  line L172 (-967.8387, 352.5) -> (-953.4049, 352.5)
  line L173 (-953.4049, 352.5) -> (-956.2917, 347.5)
  line L174 (-956.2917, 347.5) -> (-964.9519, 347.5)
  line L175 (-964.9519, 347.5) -> (-967.8387, 352.5)
  line L176 (-986.6025, 325) -> (-982.2724, 332.5)
  line L177 (-982.2724, 332.5) -> (-973.6122, 332.5)
  line L178 (-973.6122, 332.5) -> (-969.282, 325)
  line L179 (-969.282, 325) -> (-973.6122, 317.5)
  line L180 (-973.6122, 317.5) -> (-982.2724, 317.5)
  line L181 (-982.2724, 317.5) -> (-986.6025, 325)
  line L182 (-990.9327, 342.5) -> (-986.6025, 335)
  line L183 (-986.6025, 335) -> (-990.9327, 327.5)
  line L184 (-990.9327, 327.5) -> (-999.5929, 327.5)
  line L185 (-999.5929, 327.5) -> (-1003.923, 335)
  line L186 (-1003.923, 335) -> (-999.5929, 342.5)
  line L187 (-999.5929, 342.5) -> (-990.9327, 342.5)
  line L188 (-990.9327, 302.5) -> (-988.0459, 297.5)
  line L189 (-988.0459, 297.5) -> (-1002.4797, 297.5)
  line L190 (-1002.4797, 297.5) -> (-999.5929, 302.5)
  line L191 (-999.5929, 302.5) -> (-990.9327, 302.5)
  line L192 (-1037.1207, 352.5) -> (-1022.6869, 352.5)
  line L193 (-1022.6869, 352.5) -> (-1025.5737, 347.5)
  line L194 (-1025.5737, 347.5) -> (-1034.2339, 347.5)
  line L195 (-1034.2339, 347.5) -> (-1037.1207, 352.5)
  line L196 (-1042.8942, 332.5) -> (-1038.5641, 325)
  line L197 (-1038.5641, 325) -> (-1042.8942, 317.5)
  line L198 (-1042.8942, 317.5) -> (-1051.5544, 317.5)
  line L199 (-1051.5544, 317.5) -> (-1055.8846, 325)
  line L200 (-1055.8846, 325) -> (-1051.5544, 332.5)
  line L201 (-1051.5544, 332.5) -> (-1042.8942, 332.5)
  line L202 (-1060.2147, 302.5) -> (-1057.3279, 297.5)
  line L203 (-1057.3279, 297.5) -> (-1062.9423, 297.5)
  line L204 (-1062.9423, 297.5) -> (-1062.9423, 302.5)
  line L205 (-1062.9423, 302.5) -> (-1060.2147, 302.5)
  line L206 (-887.9423, 357.5) -> (-1067.9423, 357.5)
  line L207 (-1067.9423, 357.5) -> (-1067.9423, 292.5)
  line L208 (-1067.9423, 292.5) -> (-887.9423, 292.5)
  line L209 (-887.9423, 292.5) -> (-887.9423, 357.5)
  line L210 (-1067.9423, 292.5) -> (-1070.9423, 292.5)
  line L211 (-1070.9423, 292.5) -> (-1070.9423, 357.5)
  line L212 (-1070.9423, 357.5) -> (-1067.9423, 357.5)
  line L213 (-1067.9423, 357.5) -> (-1067.9423, 292.5)
  line L214 (-887.9423, 292.5) -> (-884.9423, 292.5)
  line L215 (-884.9423, 292.5) -> (-884.9423, 357.5)
  line L216 (-884.9423, 357.5) -> (-887.9423, 357.5)
  line L217 (-887.9423, 357.5) -> (-887.9423, 292.5)
  dimension "d21" = 3
  dimension "d22" = 65
  dimension "d23" = 3
  dimension "d24" = 65
  constraint horizontal L210
  constraint vertical L211
  constraint horizontal L212
  constraint vertical L213
  constraint coincident L207.end L208.start
  constraint horizontal L214
  constraint vertical L215
  constraint horizontal L216
  constraint vertical L217
  constraint coincident L208.end L209.start
  measures "d21" distance of L207.end L210.end
  measures "d22" distance of L207.end L206.end
  measures "d23" distance of L208.end L214.end
  measures "d24" distance of L208.end L206.start
extrude "Extruir3" add sketch "Boceto5" against normal blind 10 contours L209 L214 L215 L216 L217 | L207 L210 L211 L212 L213 bodies 1
sketch "Boceto6" plane through (0, 27, 0) normal (0, -1, 0) x (1, 0, 0)
  line L0 (1038.5641, 305) -> (1042.8942, 312.5)
  line L1 (1042.8942, 312.5) -> (1051.5544, 312.5)
  line L2 (1051.5544, 312.5) -> (1055.8846, 305)
  line L3 (1055.8846, 305) -> (1051.5544, 297.5)
  line L4 (1051.5544, 297.5) -> (1042.8942, 297.5)
  line L5 (1042.8942, 297.5) -> (1038.5641, 305)
  line L6 (1062.9423, 352.5) -> (1062.9423, 347.5)
  line L7 (1062.9423, 347.5) -> (1060.2147, 347.5)
  line L8 (1060.2147, 347.5) -> (1057.3279, 352.5)
  line L9 (1057.3279, 352.5) -> (1062.9423, 352.5)
  line L10 (1021.2436, 315) -> (1025.5737, 322.5)
  line L11 (1025.5737, 322.5) -> (1034.2339, 322.5)
  line L12 (1034.2339, 322.5) -> (1038.5641, 315)
  line L13 (1038.5641, 315) -> (1034.2339, 307.5)
  line L14 (1034.2339, 307.5) -> (1025.5737, 307.5)
  line L15 (1025.5737, 307.5) -> (1021.2436, 315)
  line L16 (1003.923, 345) -> (1008.2532, 352.5)
  line L17 (1008.2532, 352.5) -> (1016.9134, 352.5)
  line L18 (1016.9134, 352.5) -> (1021.2436, 345)
  line L19 (1021.2436, 345) -> (1016.9134, 337.5)
  line L20 (1016.9134, 337.5) -> (1008.2532, 337.5)
  line L21 (1008.2532, 337.5) -> (1003.923, 345)
  line L22 (969.282, 305) -> (973.6122, 312.5)
  line L23 (973.6122, 312.5) -> (982.2724, 312.5)
  line L24 (982.2724, 312.5) -> (986.6025, 305)
  line L25 (986.6025, 305) -> (982.2724, 297.5)
  line L26 (982.2724, 297.5) -> (973.6122, 297.5)
  line L27 (973.6122, 297.5) -> (969.282, 305)
  line L28 (969.282, 345) -> (973.6122, 352.5)
  line L29 (973.6122, 352.5) -> (982.2724, 352.5)
  line L30 (982.2724, 352.5) -> (986.6025, 345)
  line L31 (986.6025, 345) -> (982.2724, 337.5)
  line L32 (982.2724, 337.5) -> (973.6122, 337.5)
  line L33 (973.6122, 337.5) -> (969.282, 345)
  line L34 (934.641, 325) -> (938.9711, 332.5)
  line L35 (938.9711, 332.5) -> (947.6314, 332.5)
  line L36 (947.6314, 332.5) -> (951.9615, 325)
  line L37 (951.9615, 325) -> (947.6314, 317.5)
  line L38 (947.6314, 317.5) -> (938.9711, 317.5)
  line L39 (938.9711, 317.5) -> (934.641, 325)
  line L40 (900, 325) -> (904.3301, 332.5)
  line L41 (904.3301, 332.5) -> (912.9904, 332.5)
  line L42 (912.9904, 332.5) -> (917.3205, 325)
  line L43 (917.3205, 325) -> (912.9904, 317.5)
  line L44 (912.9904, 317.5) -> (904.3301, 317.5)
  line L45 (904.3301, 317.5) -> (900, 325)
  line L46 (900, 335) -> (895.6699, 327.5)
  line L47 (895.6699, 327.5) -> (892.9423, 327.5)
  line L48 (892.9423, 327.5) -> (892.9423, 342.5)
  line L49 (892.9423, 342.5) -> (895.6699, 342.5)
  line L50 (895.6699, 342.5) -> (900, 335)
  line L51 (900, 345) -> (904.3301, 352.5)
  line L52 (904.3301, 352.5) -> (912.9904, 352.5)
  line L53 (912.9904, 352.5) -> (917.3205, 345)
  line L54 (917.3205, 345) -> (912.9904, 337.5)
  line L55 (912.9904, 337.5) -> (904.3301, 337.5)
  line L56 (904.3301, 337.5) -> (900, 345)
  line L57 (898.5566, 352.5) -> (895.6699, 347.5)
  line L58 (895.6699, 347.5) -> (892.9423, 347.5)
  line L59 (892.9423, 347.5) -> (892.9423, 352.5)
  line L60 (892.9423, 352.5) -> (898.5566, 352.5)
  line L61 (900, 305) -> (904.3301, 312.5)
  line L62 (904.3301, 312.5) -> (912.9904, 312.5)
  line L63 (912.9904, 312.5) -> (917.3205, 305)
  line L64 (917.3205, 305) -> (912.9904, 297.5)
  line L65 (912.9904, 297.5) -> (904.3301, 297.5)
  line L66 (904.3301, 297.5) -> (900, 305)
  line L67 (934.641, 305) -> (938.9711, 312.5)
  line L68 (938.9711, 312.5) -> (947.6314, 312.5)
  line L69 (947.6314, 312.5) -> (951.9615, 305)
  line L70 (951.9615, 305) -> (947.6314, 297.5)
  line L71 (947.6314, 297.5) -> (938.9711, 297.5)
  line L72 (938.9711, 297.5) -> (934.641, 305)
  line L73 (951.9615, 335) -> (956.2917, 342.5)
  line L74 (956.2917, 342.5) -> (964.9519, 342.5)
  line L75 (964.9519, 342.5) -> (969.282, 335)
  line L76 (969.282, 335) -> (964.9519, 327.5)
  line L77 (964.9519, 327.5) -> (956.2917, 327.5)
  line L78 (956.2917, 327.5) -> (951.9615, 335)
  line L79 (953.4049, 297.5) -> (956.2917, 302.5)
  line L80 (956.2917, 302.5) -> (964.9519, 302.5)
  line L81 (964.9519, 302.5) -> (967.8387, 297.5)
  line L82 (967.8387, 297.5) -> (953.4049, 297.5)
  line L83 (988.0459, 352.5) -> (1002.4797, 352.5)
  line L84 (1002.4797, 352.5) -> (999.5929, 347.5)
  line L85 (999.5929, 347.5) -> (990.9327, 347.5)
  line L86 (990.9327, 347.5) -> (988.0459, 352.5)
  line L87 (1003.923, 305) -> (1008.2532, 312.5)
  line L88 (1008.2532, 312.5) -> (1016.9134, 312.5)
  line L89 (1016.9134, 312.5) -> (1021.2436, 305)
  line L90 (1021.2436, 305) -> (1016.9134, 297.5)
  line L91 (1016.9134, 297.5) -> (1008.2532, 297.5)
  line L92 (1008.2532, 297.5) -> (1003.923, 305)
  line L93 (1038.5641, 345) -> (1042.8942, 352.5)
  line L94 (1042.8942, 352.5) -> (1051.5544, 352.5)
  line L95 (1051.5544, 352.5) -> (1055.8846, 345)
  line L96 (1055.8846, 345) -> (1051.5544, 337.5)
  line L97 (1051.5544, 337.5) -> (1042.8942, 337.5)
  line L98 (1042.8942, 337.5) -> (1038.5641, 345)
  line L99 (1022.6869, 297.5) -> (1025.5737, 302.5)
  line L100 (1025.5737, 302.5) -> (1034.2339, 302.5)
  line L101 (1034.2339, 302.5) -> (1037.1207, 297.5)
  line L102 (1037.1207, 297.5) -> (1022.6869, 297.5)
  line L103 (1062.9423, 322.5) -> (1062.9423, 307.5)
  line L104 (1062.9423, 307.5) -> (1060.2147, 307.5)
  line L105 (1060.2147, 307.5) -> (1055.8846, 315)
  line L106 (1055.8846, 315) -> (1060.2147, 322.5)
  line L107 (1060.2147, 322.5) -> (1062.9423, 322.5)
  line L108 (1062.9423, 342.5) -> (1062.9423, 327.5)
  line L109 (1062.9423, 327.5) -> (1060.2147, 327.5)
  line L110 (1060.2147, 327.5) -> (1055.8846, 335)
  line L111 (1055.8846, 335) -> (1060.2147, 342.5)
  line L112 (1060.2147, 342.5) -> (1062.9423, 342.5)
  line L113 (1021.2436, 335) -> (1025.5737, 342.5)
  line L114 (1025.5737, 342.5) -> (1034.2339, 342.5)
  line L115 (1034.2339, 342.5) -> (1038.5641, 335)
  line L116 (1038.5641, 335) -> (1034.2339, 327.5)
  line L117 (1034.2339, 327.5) -> (1025.5737, 327.5)
  line L118 (1025.5737, 327.5) -> (1021.2436, 335)
  line L119 (1003.923, 325) -> (1008.2532, 332.5)
  line L120 (1008.2532, 332.5) -> (1016.9134, 332.5)
  line L121 (1016.9134, 332.5) -> (1021.2436, 325)
  line L122 (1021.2436, 325) -> (1016.9134, 317.5)
  line L123 (1016.9134, 317.5) -> (1008.2532, 317.5)
  line L124 (1008.2532, 317.5) -> (1003.923, 325)
  line L125 (986.6025, 315) -> (990.9327, 322.5)
  line L126 (990.9327, 322.5) -> (999.5929, 322.5)
  line L127 (999.5929, 322.5) -> (1003.923, 315)
  line L128 (1003.923, 315) -> (999.5929, 307.5)
  line L129 (999.5929, 307.5) -> (990.9327, 307.5)
  line L130 (990.9327, 307.5) -> (986.6025, 315)
  line L131 (951.9615, 315) -> (956.2917, 322.5)
  line L132 (956.2917, 322.5) -> (964.9519, 322.5)
  line L133 (964.9519, 322.5) -> (969.282, 315)
  line L134 (969.282, 315) -> (964.9519, 307.5)
  line L135 (964.9519, 307.5) -> (956.2917, 307.5)
  line L136 (956.2917, 307.5) -> (951.9615, 315)
  line L137 (934.641, 345) -> (938.9711, 352.5)
  line L138 (938.9711, 352.5) -> (947.6314, 352.5)
  line L139 (947.6314, 352.5) -> (951.9615, 345)
  line L140 (951.9615, 345) -> (947.6314, 337.5)
  line L141 (947.6314, 337.5) -> (938.9711, 337.5)
  line L142 (938.9711, 337.5) -> (934.641, 345)
  line L143 (917.3205, 315) -> (921.6506, 322.5)
  line L144 (921.6506, 322.5) -> (930.3109, 322.5)
  line L145 (930.3109, 322.5) -> (934.641, 315)
  line L146 (934.641, 315) -> (930.3109, 307.5)
  line L147 (930.3109, 307.5) -> (921.6506, 307.5)
  line L148 (921.6506, 307.5) -> (917.3205, 315)
  line L149 (892.9423, 307.5) -> (892.9423, 322.5)
  line L150 (892.9423, 322.5) -> (895.6699, 322.5)
  line L151 (895.6699, 322.5) -> (900, 315)
  line L152 (900, 315) -> (895.6699, 307.5)
  line L153 (895.6699, 307.5) -> (892.9423, 307.5)
  line L154 (917.3205, 335) -> (921.6506, 342.5)
  line L155 (921.6506, 342.5) -> (930.3109, 342.5)
  line L156 (930.3109, 342.5) -> (934.641, 335)
  line L157 (934.641, 335) -> (930.3109, 327.5)
  line L158 (930.3109, 327.5) -> (921.6506, 327.5)
  line L159 (921.6506, 327.5) -> (917.3205, 335)
  line L160 (918.7639, 352.5) -> (933.1976, 352.5)
  line L161 (933.1976, 352.5) -> (930.3109, 347.5)
  line L162 (930.3109, 347.5) -> (921.6506, 347.5)
  line L163 (921.6506, 347.5) -> (918.7639, 352.5)
  line L164 (892.9423, 297.5) -> (892.9423, 302.5)
  line L165 (892.9423, 302.5) -> (895.6699, 302.5)
  line L166 (895.6699, 302.5) -> (898.5566, 297.5)
  line L167 (898.5566, 297.5) -> (892.9423, 297.5)
  line L168 (918.7639, 297.5) -> (921.6506, 302.5)
  line L169 (921.6506, 302.5) -> (930.3109, 302.5)
  line L170 (930.3109, 302.5) -> (933.1976, 297.5)
  line L171 (933.1976, 297.5) -> (918.7639, 297.5)
  line L172 (953.4049, 352.5) -> (967.8387, 352.5)
  line L173 (967.8387, 352.5) -> (964.9519, 347.5)
  line L174 (964.9519, 347.5) -> (956.2917, 347.5)
  line L175 (956.2917, 347.5) -> (953.4049, 352.5)
  line L176 (982.2724, 332.5) -> (986.6025, 325)
  line L177 (986.6025, 325) -> (982.2724, 317.5)
  line L178 (982.2724, 317.5) -> (973.6122, 317.5)
  line L179 (973.6122, 317.5) -> (969.282, 325)
  line L180 (969.282, 325) -> (973.6122, 332.5)
  line L181 (973.6122, 332.5) -> (982.2724, 332.5)
  line L182 (986.6025, 335) -> (990.9327, 342.5)
  line L183 (990.9327, 342.5) -> (999.5929, 342.5)
  line L184 (999.5929, 342.5) -> (1003.923, 335)
  line L185 (1003.923, 335) -> (999.5929, 327.5)
  line L186 (999.5929, 327.5) -> (990.9327, 327.5)
  line L187 (990.9327, 327.5) -> (986.6025, 335)
  line L188 (988.0459, 297.5) -> (990.9327, 302.5)
  line L189 (990.9327, 302.5) -> (999.5929, 302.5)
  line L190 (999.5929, 302.5) -> (1002.4797, 297.5)
  line L191 (1002.4797, 297.5) -> (988.0459, 297.5)
  line L192 (1022.6869, 352.5) -> (1037.1207, 352.5)
  line L193 (1037.1207, 352.5) -> (1034.2339, 347.5)
  line L194 (1034.2339, 347.5) -> (1025.5737, 347.5)
  line L195 (1025.5737, 347.5) -> (1022.6869, 352.5)
  line L196 (1038.5641, 325) -> (1042.8942, 332.5)
  line L197 (1042.8942, 332.5) -> (1051.5544, 332.5)
  line L198 (1051.5544, 332.5) -> (1055.8846, 325)
  line L199 (1055.8846, 325) -> (1051.5544, 317.5)
  line L200 (1051.5544, 317.5) -> (1042.8942, 317.5)
  line L201 (1042.8942, 317.5) -> (1038.5641, 325)
  line L202 (1057.3279, 297.5) -> (1060.2147, 302.5)
  line L203 (1060.2147, 302.5) -> (1062.9423, 302.5)
  line L204 (1062.9423, 302.5) -> (1062.9423, 297.5)
  line L205 (1062.9423, 297.5) -> (1057.3279, 297.5)
  line L206 (1067.9423, 357.5) -> (887.9423, 357.5)
  line L207 (887.9423, 357.5) -> (887.9423, 292.5)
  line L208 (887.9423, 292.5) -> (1067.9423, 292.5)
  line L209 (1067.9423, 292.5) -> (1067.9423, 357.5)
  line L210 (1067.9423, 292.5) -> (1064.9423, 292.5)
  line L211 (1064.9423, 292.5) -> (1064.9423, 357.5)
  line L212 (1064.9423, 357.5) -> (1067.9423, 357.5)
  line L213 (1067.9423, 357.5) -> (1067.9423, 292.5)
  line L214 (887.9423, 292.5) -> (890.9423, 292.5)
  line L215 (890.9423, 292.5) -> (890.9423, 357.5)
  line L216 (890.9423, 357.5) -> (887.9423, 357.5)
  line L217 (887.9423, 357.5) -> (887.9423, 292.5)
  dimension "d27" = 3
  dimension "d28" = 3
  dimension "d29" = 65
  constraint horizontal L210
  constraint vertical L211
  constraint horizontal L212
  constraint vertical L213
  constraint coincident L208.end L209.start
  constraint horizontal L214
  constraint vertical L215
  constraint horizontal L216
  constraint vertical L217
  constraint coincident L207.end L208.start
  measures "d27" distance of L208.end L210.end
  measures "d28" distance of L207.end L214.end
  measures "d29" distance of L207.end L206.end
extrude "Extruir4" add sketch "Boceto6" along normal blind 77.5 separate body contours L206 L208 L209 L210 L211 L212 L213 | L206 L207 L208 L214 L215 L216 L217 makes body 2 at (1067.9423, 1.1667, 314.1667) makes body 3 at (890.9423, 1.1667, 314.1667)